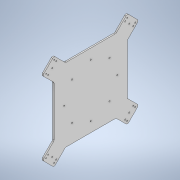
# Autodesk Inventor part: Frame
Saved by Autodesk Inventor 2022 (Build 260153000, 153)
## iProperties
Created: 2022-02-12
Part Number: Frame
Material: Generic
Document SubType Name: Modeling
Designer: ultra
Density: 1 g/cm^3
Appearance: Default
Author: ultra
Autodesk Inventor part; units mm, degrees
ref_plane "YZ Plane" through (0, 0, 0) normal (1, 0, 0) x (0, 1, 0)
ref_plane "XZ Plane" through (0, 0, 0) normal (0, 1, 0) x (-1, 0, 0)
ref_plane "XY Plane" through (0, 0, 0) normal (0, 0, 1) x (1, 0, 0)
sketch "Sketch1" plane through (0, 0, 0) normal (1, 0, 0) x (0, 1, 0)
  line L0 (0, 0) -> (321.6656, 0)
  line L1 (321.6656, 0) -> (321.6656, 321.6656)
  line L2 (321.6656, 321.6656) -> (0, 321.6656)
  line L3 (0, 321.6656) -> (0, 0)
  dimension "d0" = 321.6656
  dimension "d1" = 321.6656
  constraints: 8 end point, 2 parallel, 1 horizontal, 1 perpendicular
  measures "d0" distance of L2.end L1.end
  measures "d1" distance of L1.end L0.end
extrude "Extrusion1" add sketch "Sketch1" along normal blind 4.7752
sketch "Sketch3" plane through (0, 0, 0) normal (-1, 0, 0) x (0, 0, 1)
  line L0 (0, 321.6656) -> (321.6656, 321.6656) projected
  line L1 (321.6656, 321.6656) -> (321.6656, 0) projected
  line L2 (0, 321.6656) -> (321.6656, 321.6656) projected
  line L3 (321.6656, 321.6656) -> (283.5656, 321.6656)
  line L4 (283.5656, 321.6656) -> (283.5656, 283.5656)
  line L5 (283.5656, 283.5656) -> (321.6656, 283.5656)
  line L6 (321.6656, 283.5656) -> (321.6656, 321.6656)
  line L7 (321.6656, 321.6656) -> (321.6656, 0) projected
  line L8 (321.6656, 0) -> (283.5656, 0)
  line L9 (283.5656, 0) -> (283.5656, 38.1)
  line L10 (283.5656, 38.1) -> (321.6656, 38.1)
  line L11 (321.6656, 38.1) -> (321.6656, 0)
  line L12 (321.6656, 0) -> (0, 0) projected
  line L13 (0, 0) -> (38.1, 0)
  line L14 (38.1, 0) -> (38.1, 38.1)
  line L15 (38.1, 38.1) -> (0, 38.1)
  line L16 (0, 38.1) -> (0, 0)
  line L17 (0, 321.6656) -> (38.1, 321.6656)
  line L18 (38.1, 321.6656) -> (38.1, 283.5656)
  line L19 (38.1, 283.5656) -> (0, 283.5656)
  line L20 (0, 283.5656) -> (0, 321.6656)
  line L21 (283.5656, 321.6656) -> (38.1, 321.6656)
  line L22 (38.1, 321.6656) -> (38.1, 283.5656)
  line L23 (38.1, 283.5656) -> (283.5656, 283.5656)
  line L24 (283.5656, 283.5656) -> (283.5656, 321.6656)
  line L25 (321.6656, 283.5656) -> (283.5656, 283.5656)
  line L26 (283.5656, 283.5656) -> (283.5656, 38.1)
  line L27 (283.5656, 38.1) -> (321.6656, 38.1)
  line L28 (321.6656, 38.1) -> (321.6656, 283.5656)
  line L29 (38.1, 38.1) -> (0, 38.1)
  line L30 (0, 38.1) -> (0, 283.5656)
  line L31 (0, 283.5656) -> (38.1, 283.5656)
  line L32 (38.1, 283.5656) -> (38.1, 38.1)
  line L33 (38.1, 38.1) -> (283.5656, 38.1)
  line L34 (283.5656, 38.1) -> (283.5656, 0)
  line L35 (283.5656, 0) -> (38.1, 0)
  line L36 (38.1, 0) -> (38.1, 38.1)
  line L37 (321.6656, 283.5656) -> (283.5656, 245.4656)
  line L38 (321.6656, 283.5656) -> (375.5471, 283.5656) construction
  line L39 (283.5656, 245.4656) -> (283.5656, 321.6656)
  line L40 (283.5656, 321.6656) -> (245.4656, 283.5656)
  line L41 (283.5656, 321.6656) -> (337.4471, 321.6656) construction
  line L42 (38.1, 321.6656) -> (76.2, 283.5656)
  line L43 (38.1, 321.6656) -> (91.9815, 321.6656) construction
  line L44 (0, 283.5656) -> (38.1, 245.4656)
  line L45 (0, 283.5656) -> (53.8815, 283.5656) construction
  line L46 (0, 38.1) -> (38.1, 76.2)
  line L47 (0, 38.1) -> (53.8815, 38.1) construction
  line L48 (38.1, 0) -> (76.2, 38.1)
  line L49 (38.1, 0) -> (91.9815, 0) construction
  line L50 (321.6656, 38.1) -> (283.5656, 76.2)
  line L51 (321.6656, 38.1) -> (375.5471, 38.1) construction
  line L52 (283.5656, 0) -> (245.4656, 38.1)
  line L53 (283.5656, 0) -> (337.4471, 0) construction
  dimension "d14" = 38.1
  dimension "d15" = 38.1
  dimension "d16" = 38.1
  dimension "d17" = 38.1
  dimension "d18" = 38.1
  dimension "d19" = 38.1
  dimension "d20" = 38.1
  dimension "d21" = 135
  dimension "d22" = 135
  dimension "d25" = 45
  dimension "d26" = 45
  dimension "d27" = 45
  dimension "d28" = 45
  dimension "d29" = 135
  dimension "d30" = 135
  constraints: 98 end point, 16 horizontal, 16 parallel, 9 point on line, 8 equal length, 8 perpendicular, 1 collinear
  measures "d14" distance of L5.end L4.end
  measures "d15" distance of L4.end L3.end
  measures "d16" distance of L8.end L9.end
  measures "d17" distance of L15.end L14.end
  measures "d18" distance of L14.end L13.end
  measures "d19" distance of L18.end L19.end
  measures "d20" distance of L17.end L18.end
  measures "d21" angle of L37 L38
  measures "d22" angle of L40 L41
  measures "d25" angle of L42 L43
  measures "d26" angle of L44 L45
  measures "d27" angle of L47 L46
  measures "d28" angle of L49 L48
  measures "d29" angle of L51 L50
  measures "d30" angle of L53 L52
extrude "Extrusion4" cut sketch "Sketch3" against normal blind 4.7752 contours L0 L40 L23 L42 | L44 L32 L46 L30 | L1 L50 L26 L37 | L48 L33 L52 L12
sketch "Sketch4" plane through (0, 0, 0) normal (-1, 0, 0) x (0, 0, 1)
  line L0 (321.6656, 0) -> (283.5656, 0) projected
  line L1 (321.6656, 38.1) -> (321.6656, 0) projected
  line L2 (321.6656, 321.6656) -> (321.6656, 283.5656) projected
  line L3 (283.5656, 321.6656) -> (321.6656, 321.6656) projected
  line L4 (0, 321.6656) -> (38.1, 321.6656) projected
  line L5 (0, 283.5656) -> (0, 321.6656) projected
  line L6 (0, 0) -> (0, 38.1) projected
  line L7 (38.1, 0) -> (0, 0) projected
  line L8 (245.4656, 283.5656) -> (283.5656, 321.6656) projected
  line L9 (283.5656, 321.6656) -> (321.6656, 283.5656)
  line L10 (0, 283.5656) -> (0, 321.6656) projected
  line L11 (38.1, 321.6656) -> (0, 283.5656)
  line L12 (0, 38.1) -> (38.1, 0)
  line L13 (283.5656, 0) -> (321.6656, 38.1)
  constraints: 8 end point, 2 perpendicular, 1 point on line
extrude "Extrusion5" cut sketch "Sketch4" against normal blind 4.7752
fillet "Fillet1" radius 6.35 16 edges at (2.3876, 283.5656, 0) (2.3876, 321.6656, 38.1) (2.3876, 38.1, 0) (2.3876, 76.2, 38.1) (2.3876, 0, 38.1) (2.3876, 283.5656, 76.2) (2.3876, 283.5656, 245.4656) (2.3876, 321.6656, 283.5656) (2.3876, 283.5656, 321.6656) (2.3876, 76.2, 283.5656) (2.3876, 245.4656, 283.5656) (2.3876, 0, 283.5656) (2.3876, 38.1, 321.6656) (2.3876, 38.1, 76.2) (2.3876, 38.1, 245.4656) (2.3876, 245.4656, 38.1)
sketch "Sketch6" plane through (0, 0, 0) normal (-1, 0, 0) x (0, 0, 1)
  circle A0 centre (-6.7619, -6.7309) radius 6.35
  circle A1 centre (71.9016, 17.9648) radius 6.35
  circle A2 centre (-24.7224, -24.6915) radius 6.35
  circle A3 centre (18.3502, 71.9326) radius 6.35
  circle A4 centre (39.0622, 11.5317) radius 2.159
  circle A5 centre (45.6554, 18.406) radius 2.159
  circle A6 centre (18.4365, 45.0628) radius 2.159
  circle A7 centre (32.185, 31.8764) radius 2.159
  circle A8 centre (11.8433, 38.1885) radius 2.159
  arc A9 (79.2947, 3.1748) -> (87.7766, 8.3381) centre (85.2874, 2.8788) ccw
  line L0 (87.7766, 28.6693) -> (87.7766, 8.3381)
  arc A10 (87.7766, 28.6693) -> (79.2947, 33.8326) centre (85.2874, 34.1286) ccw
  line L1 (40.1516, 33.8326) -> (79.2947, 33.8326)
  arc A11 (33.8016, 40.1826) -> (40.1516, 33.8326) centre (40.1516, 40.1826) ccw
  line L2 (33.8016, 79.3257) -> (33.8016, 40.1826)
  arc A12 (33.8016, 79.3257) -> (28.6383, 87.8076) centre (34.0976, 85.3184) ccw
  line L3 (28.6383, 87.8076) -> (8.3071, 87.8076)
  arc A13 (8.3071, 87.8076) -> (3.1438, 79.3257) centre (2.8478, 85.3184) ccw
  line L4 (3.1438, 27.4834) -> (3.1438, 79.3257)
  arc A14 (1.284, 22.9933) -> (3.1438, 27.4834) centre (-3.2062, 27.4834) ccw
  line L5 (-40.7893, -19.08) -> (1.284, 22.9933)
  arc A15 (-28.7596, -43.1049) -> (-19.111, -40.7583) centre (-23.1391, -45.2051) ccw
  line L6 (22.9623, 1.3149) -> (-19.111, -40.7583)
  arc A16 (27.4524, 3.1748) -> (22.9623, 1.3149) centre (27.4524, -3.1752) ccw
  line L7 (79.2947, 3.1748) -> (27.4524, 3.1748)
  circle A17 centre (85.2874, 34.1286) radius 2.95
  circle A18 centre (2.8478, 85.3184) radius 2.95
  circle A19 centre (-23.1391, -45.2051) radius 2.95
  circle A20 centre (85.2874, 2.8788) radius 2.95
  circle A21 centre (34.0976, 85.3184) radius 2.95
  point P0 (0, 0)
  point P1 (36.9766, 87.8076)
  dimension "d65" = 4.318
  constraints: 22 centre point, 16 end point, 16 point on circle
  measures "d65" diameter of A8
extrude "Extrusion7" cut sketch "Sketch6" against normal blind 25.4 contours A4 | A5 | A6 | A7 | A8
sketch "Sketch7" plane through (4.7752, 0, 0) normal (1, 0, 0) x (0, 0, -1)
  circle A0 centre (-31.8764, 289.4806) radius 2.159
  circle A1 centre (-11.5317, 282.6034) radius 2.159
  circle A2 centre (-38.1885, 309.8223) radius 2.159
  circle A3 centre (-18.406, 276.0102) radius 2.159
  circle A4 centre (-45.0628, 303.2291) radius 2.159
  circle A5 centre (-81.9118, 239.7538) radius 19.05
  line L0 (-38.1, 78.8303) -> (-38.1, 242.8353)
  arc A6 (-36.2401, 247.3255) -> (-38.1, 242.8353) centre (-31.75, 242.8353) ccw
  line L1 (-36.2401, 247.3255) -> (-4.4901, 279.0755)
  arc A7 (-4.4901, 279.0755) -> (-4.4901, 288.0557) centre (-8.9803, 283.5656) ccw
  line L2 (-4.4901, 288.0557) -> (-33.6099, 317.1755)
  arc A8 (-33.6099, 317.1755) -> (-42.5901, 317.1755) centre (-38.1, 312.6853) ccw
  line L3 (-42.5901, 317.1755) -> (-74.3401, 285.4255)
  arc A9 (-78.8303, 283.5656) -> (-74.3401, 285.4255) centre (-78.8303, 289.9156) ccw
  line L4 (-78.8303, 283.5656) -> (-242.8353, 283.5656)
  point P0 (0, 0)
  point P1 (-61.0348, 364.3954)
  constraints: 10 centre point, 10 end point, 8 point on circle
extrude "Extrusion8" cut sketch "Sketch7" against normal blind 25.4 contours A0 | A1 | A2 | A3 | A4
sketch "Sketch8" plane through (4.7752, 0, 0) normal (1, 0, 0) x (0, 0, -1)
  circle A0 centre (-289.7892, 32.185) radius 2.159
  circle A1 centre (-310.1339, 39.0622) radius 2.159
  circle A2 centre (-276.6028, 18.4365) radius 2.159
  circle A3 centre (-303.2596, 45.6554) radius 2.159
  circle A4 centre (-283.4771, 11.8433) radius 2.159
  circle A5 centre (-289.4806, 289.7892) radius 2.159
  circle A6 centre (-282.6034, 310.1339) radius 2.159
  circle A7 centre (-309.8223, 283.4771) radius 2.159
  circle A8 centre (-276.0102, 303.2596) radius 2.159
  circle A9 centre (-303.2291, 276.6028) radius 2.159
  circle A10 centre (-239.7538, 81.9118) radius 19.05
  circle A11 centre (-239.7538, 239.7538) radius 19.05
  line L0 (-78.8303, 283.5656) -> (-242.8353, 283.5656)
  arc A12 (-247.3255, 285.4255) -> (-242.8353, 283.5656) centre (-242.8353, 289.9156) ccw
  line L1 (-247.3255, 285.4255) -> (-279.0755, 317.1755)
  arc A13 (-279.0755, 317.1755) -> (-288.0557, 317.1755) centre (-283.5656, 312.6853) ccw
  line L2 (-288.0557, 317.1755) -> (-317.1755, 288.0557)
  arc A14 (-317.1755, 288.0557) -> (-317.1755, 279.0755) centre (-312.6853, 283.5656) ccw
  line L3 (-317.1755, 279.0755) -> (-285.4255, 247.3255)
  arc A15 (-283.5656, 242.8353) -> (-285.4255, 247.3255) centre (-289.9156, 242.8353) ccw
  line L4 (-283.5656, 242.8353) -> (-283.5656, 78.8303)
  arc A16 (-285.4255, 74.3401) -> (-283.5656, 78.8303) centre (-289.9156, 78.8303) ccw
  line L5 (-285.4255, 74.3401) -> (-317.1755, 42.5901)
  arc A17 (-317.1755, 42.5901) -> (-317.1755, 33.6099) centre (-312.6853, 38.1) ccw
  line L6 (-317.1755, 33.6099) -> (-288.0557, 4.4901)
  arc A18 (-288.0557, 4.4901) -> (-279.0755, 4.4901) centre (-283.5656, 8.9803) ccw
  line L7 (-279.0755, 4.4901) -> (-247.3255, 36.2401)
  arc A19 (-242.8353, 38.1) -> (-247.3255, 36.2401) centre (-242.8353, 31.75) ccw
  line L8 (-242.8353, 38.1) -> (-78.8303, 38.1)
  point P0 (0, 0)
  point P1 (-321.6656, 321.6656)
  constraints: 20 centre point, 18 end point, 16 point on circle
extrude "Extrusion9" cut sketch "Sketch8" against normal blind 25.4 contours A0 | A1 | A2 | A3 | A4 | A5 | A6 | A7 | A8 | A9
sketch "Sketch9" plane through (4.7752, 0, 0) normal (1, 0, 0) x (0, 0, -1)
  circle A0 centre (-160.8328, 160.8328) radius 19.05
  circle A1 centre (-160.8328, 160.8328) radius 88.9
  circle A2 centre (-160.8328, 249.7328) radius 2.032
  circle A3 centre (-223.6946, 223.6946) radius 2.032
  circle A4 centre (-249.7328, 160.8328) radius 2.032
  circle A5 centre (-223.6946, 97.971) radius 2.032
  circle A6 centre (-160.8328, 71.9328) radius 2.032
  circle A7 centre (-97.971, 97.971) radius 2.032
  circle A8 centre (-71.9328, 160.8328) radius 2.032
  circle A9 centre (-97.971, 223.6946) radius 2.032
  point P0 (0, 0)
  dimension "d54" = 177.8
  dimension "d53" = 38.1
  dimension "d55" = 4.064
  dimension "d61" = 360
  constraints: 9 centre point, 1 coincident, 1 vertical alignment, 19 other
  measures "d53" diameter of A0
  measures "d55" diameter of A2
extrude "Extrusion10" cut sketch "Sketch9" against normal blind 25.4 contours A1 A8 | A1 A8 | A9 A1 | A1 A9 | A7 A1 | A1 A7 | A2 A1 | A1 A2 | A6 A1 | A1 A6 | A3 A1 | A1 A3 | A5 A1 | A1 A5 | A4 A1 | A1 A4
body "Solid1"
